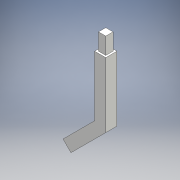
# Autodesk Inventor part: Stalk_v2
Saved by Autodesk Inventor 2016 (Build 200138000, 138)
## iProperties
Created: 2015-11-02
Part Number: Stalk_v2
Material: Generic
Document SubType Name: Modeling
Designer: Jared
Density: 1 g/cm^3
Appearance: Default
Author: Jared
Autodesk Inventor part; units mm, degrees
ref_plane "YZ Plane" through (0, 0, 0) normal (1, 0, 0) x (0, 1, 0)
ref_plane "XZ Plane" through (0, 0, 0) normal (0, 1, 0) x (-1, 0, 0)
ref_plane "XY Plane" through (0, 0, 0) normal (0, 0, 1) x (1, 0, 0)
sketch "Sketch1" plane through (0, 0, 0) normal (0, 1, 0) x (-1, 0, 0)
  line L0 (0, 0) -> (-10, 0)
  line L1 (-10, 0) -> (-10, -54)
  line L2 (0, -54) -> (0, 0)
  line L3 (0, -54) -> (28.2843, -82.2843)
  line L4 (0, -54) -> (40, -54) construction
  line L5 (28.2843, -82.2843) -> (21.2132, -89.3553)
  line L6 (21.2132, -89.3553) -> (-10, -58.1421)
  line L7 (-10, -58.1421) -> (-10, -54)
  constraints: 16 end point, 3 perpendicular, 2 horizontal, 1 equal length, 1 parallel, 1 vertical
extrude "Extrusion1" add sketch "Sketch1" along normal blind 10
sketch "Sketch2" plane through (0, 0, 0) normal (0, 0, 1) x (1, 0, 0)
  line L0 (1.75, 1.75) -> (8.25, 1.75)
  line L1 (8.25, 1.75) -> (8.25, 8.25)
  line L2 (8.25, 8.25) -> (1.75, 8.25)
  line L3 (1.75, 8.25) -> (1.75, 1.75)
  point P0 (0, 0)
  constraints: 8 end point, 2 parallel, 1 horizontal, 1 perpendicular
extrude "Extrusion2" add sketch "Sketch2" along normal blind 15
sketch "Sketch3" plane through (-28.2843, 0, -82.2843) normal (-0.7071, 0, -0.7071) x (-0.7071, 0, 0.7071)
  line L0 (-2.25, 2.25) -> (-7.75, 2.25)
  line L1 (-7.75, 2.25) -> (-7.75, 7.75)
  line L2 (-7.75, 7.75) -> (-2.25, 7.75)
  line L3 (-2.25, 7.75) -> (-2.25, 2.25)
  point P0 (38.1838, 0)
  constraints: 8 end point, 2 parallel, 1 horizontal, 1 perpendicular
extrude "Extrusion3" cut sketch "Sketch3" against normal blind 10
body "Solid1"
